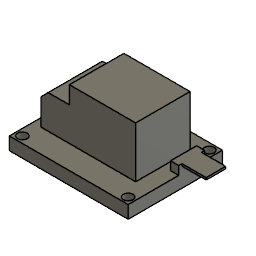
rele (Autodesk Fusion 360 design; units mm, degrees)
part number: 2026-03-25-11-49-12-979
Autodesk Fusion 360 part; units mm, degrees
sketch "Boceto1" plane through (0, 0, 0) normal (0, 1, 0) x (1, 0, 0)
  line L0 (16.7, -13.25) -> (-16.7, -13.25)
  line L1 (-16.7, -13.25) -> (-16.7, 13.25)
  line L2 (-16.7, 13.25) -> (16.7, 13.25)
  line L3 (16.7, 13.25) -> (16.7, -13.25)
  line L4 (16.7, -13.25) -> (-16.7, 13.25) construction
  line L5 (-16.7, -13.25) -> (16.7, 13.25) construction
  line L6 (-14.4, 8.65) -> (12.2, 8.65)
  line L7 (12.2, 8.65) -> (12.2, -6.65)
  line L8 (12.2, -6.65) -> (-14.4, -6.65)
  line L9 (-14.4, -6.65) -> (-14.4, 8.65)
  line L10 (-6.4, 8.65) -> (-6.4, -6.65)
  circle A0 centre (-14.85, 11.4) radius 1.35
  circle A1 centre (14.85, 11.4) radius 1.35
  circle A2 centre (14.85, -11.4) radius 1.35
  circle A3 centre (-14.85, -11.4) radius 1.35
  line L11 (14.4, 8.25) -> (16.7, 8.25)
  line L12 (16.7, 8.25) -> (16.7, 0.95)
  line L13 (16.7, 0.95) -> (14.4, 0.95)
  line L14 (14.4, 0.95) -> (14.4, 8.25)
  dimension "d1" = 33.4
  dimension "d2" = 26.5
  dimension "d3" = 26.6
  dimension "d4" = 15.3
  dimension "d5" = 4.6
  dimension "d6" = 4.5
  dimension "d8" = 8
  dimension "d16" = 2.7
  dimension "d17" = 1.85
  dimension "d18" = 1.85
  dimension "d19" = 1.85
  dimension "d20" = 1.85
  dimension "d21" = 5
  dimension "d22" = 2.3
  dimension "d23" = 7.3
  constraint horizontal L0
  constraint perpendicular L0 L1
  constraint parallel L0 L2
  constraint parallel L1 L3
  constraint coincident L4 origin
  constraint coincident L5 origin
  constraint horizontal L6
  constraint vertical L7
  constraint horizontal L8
  constraint vertical L9
  constraint coincident L6 L10.start
  constraint coincident L8 L10.end
  constraint perpendicular L8 L10
  constraint equal A0 A1
  constraint equal A1 A2
  constraint equal A2 A3
  constraint horizontal A0.centre A1.centre
  constraint vertical A0.centre A3.centre
  constraint horizontal A2.centre A3.centre
  constraint vertical A1.centre A2.centre
  constraint horizontal L11
  constraint vertical L12
  constraint horizontal L13
  constraint vertical L14
  constraint collinear L3 L12
  measures "d1" distance of L1.end L2.end
  measures "d2" distance of L0.start L2.end
  measures "d3" distance of L7 L9
  measures "d4" distance of L6.end L7.end
  measures "d5" distance of L2 L6
  measures "d6" distance of L3 L7
  measures "d8" distance of L9 L10
  measures "d16" diameter of A0
  measures "d17" distance of L2 A0.centre
  measures "d18" distance of L1 A0.centre
  measures "d19" distance of L3 A1.centre
  measures "d20" distance of L0 A2.centre
  measures "d21" distance of L2 L11
  measures "d22" distance of L12 L14
  measures "d23" distance of L11.start L13.end
extrude "Extruir1" add sketch "Boceto1" along normal blind 3.6 contours L0 L1 L2 L3 L11 L13 L14 | L3 L11 L12 L13 L14 | L6 L8 L9 L10 | L6 L7 L8 L10
extrude "Extruir2" add sketch "Boceto1" along normal blind 17.9 contours L6 L7 L8 L10
extrude "Extruir3" add sketch "Boceto1" along normal blind 13 contours L6 L8 L9 L10
chamfer "Chaflán1" distance 2 angle 45 1 edges at (-14.4, 13, -1)
extrude "Extruir4" add sketch "Boceto1" along normal blind 6 contours L3 L11 L12 L13 L14
sketch "Boceto2" plane through (16.7, 0, 0) normal (1, 0, 0) x (0, 0, -1)
  line L0 (0.95, 3.6) -> (-13.25, 3.6)
  line L1 (-13.25, 3.6) -> (-13.25, 0)
  line L2 (-13.25, 0) -> (13.25, 0)
  line L3 (13.25, 0) -> (13.25, 3.6)
  line L4 (13.25, 3.6) -> (8.25, 3.6)
  line L5 (8.25, 3.6) -> (8.25, 6)
  line L6 (8.25, 6) -> (0.95, 6)
  line L7 (0.95, 6) -> (0.95, 3.6)
  line L8 (1.85, 6) -> (7.35, 6)
  line L9 (7.35, 6) -> (7.35, 5.4)
  line L10 (7.35, 5.4) -> (1.85, 5.4)
  line L11 (1.85, 5.4) -> (1.85, 6)
  point P0 (4.6, 6)
  point P1 (4.6, 6)
  dimension "d26" = 0.6
  dimension "d27" = 5.5
  constraint horizontal L8
  constraint vertical L9
  constraint horizontal L10
  constraint vertical L11
  constraint midpoint L8 P1
  constraint midpoint L6 P1
  constraint vertical P1 P0
  constraint coincident P1 P0
  measures "d26" distance of L8.end L9.end
  measures "d27" distance of L8.start L8.end
extrude "Extruir5" add sketch "Boceto2" along normal blind 6.8 contours L6 L8 L9 L10 L11
equation "d9 = 1.2 mm + 2.4 mm"
equation "d11 = 16.7 mm + 1.2 mm"
equation "d17 = 0.5 mm + ( ( 2.7 / 2 ) * 1 mm )"
equation "d18 = 0.5 mm + ( ( 2.7 / 2 ) * 1 mm )"
equation "d19 = 0.5 mm + ( ( 2.7 / 2 ) * 1 mm )"
equation "d20 = 0.5 mm + ( ( 2.7 / 2 ) * 1 mm )"
